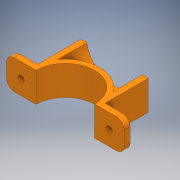
# Autodesk Inventor part: Motor Mount C-Clamp Base
Saved by Autodesk Inventor 2018 (Build 220112000, 112)
## iProperties
Created: 2018-01-11
Part Number: Motor Mount C-Clamp Base
Material: Generic
Document SubType Name: Modeling
Designer: Moochster
Density: 1 g/cm^3
Appearance: Orange
Author: Moochster
Autodesk Inventor part; units mm, degrees
ref_plane "YZ Plane" through (0, 0, 0) normal (1, 0, 0) x (0, 1, 0)
ref_plane "XY Plane" through (0, 0, 0) normal (0, 0, 1) x (1, 0, 0)
sketch "Sketch1" plane through (0, 0, 0) normal (0, 0, 1) x (1, 0, 0)
  arc A0 (14.865, 0) -> (-14.865, 0) centre (0, 0) ccw
  arc A1 (17.1039, 3) -> (-17.1039, 3) centre (0, 0) ccw
  line L0 (-17.1039, 3) -> (-29.865, 3)
  line L1 (-29.865, 3) -> (-29.865, 0)
  line L2 (-29.865, 0) -> (-14.865, 0)
  line L3 (14.865, 0) -> (29.865, 0)
  line L4 (29.865, 0) -> (29.865, 3)
  line L5 (29.865, 3) -> (17.1039, 3)
  dimension "d0" = 3
  dimension "d1" = 14.865
  dimension "d2" = 2.5
  dimension "d3" = 15
  constraints: 12 end point, 4 horizontal, 4 point on circle, 3 horizontal alignment, 2 centre point, 2 coincident, 2 perpendicular, 1 collinear, 1 concentric
  measures "d0" distance of L3.end L4.end
  measures "d1" radius of A0
  measures "d2" radial gap between concentric circles of A0 A1
  measures "d3" distance of L3.start L3.end
extrude "Extrusion1" add sketch "Sketch1" along normal blind 15
sketch "Sketch2" plane through (-29.865, 0, 0) normal (0, -1, 0) x (1, 0, 0)
  line L0 (0, 15) -> (15, 15) projected
  line L1 (0, 0) -> (0, 15) projected
  point P0 (29.865, 0)
  point P1 (7.5, 7.5)
  point P2 (7.5, 15)
  point P3 (0, 7.5)
  constraints: 2 midpoint, 1 horizontal alignment, 1 vertical alignment
hole "Hole1" at (-22.365, 0, 7.5) direction (0, 1, 0) diameter 3 end through all
mirror "Mirror1" about plane through (0, 0, 0) normal (1, 0, 0) of "Hole1"
ref_plane "Work Plane1" through (0, 25, 0) normal (0, 1, 0) x (-1, 0, 0)
sketch "Sketch3" plane through (0, 25, 0) normal (0, 1, 0) x (-1, 0, 0)
  line L0 (-17.1039, 0) -> (17.1039, 0) projected
  line L1 (-17.1039, 0) -> (-17.1039, 15) projected
  line L2 (17.1039, 0) -> (17.1039, 15) projected
  line L3 (-17.1039, 15) -> (-14.1039, 15)
  line L4 (17.1039, 15) -> (14.1039, 15)
  arc A0 (-14.1039, 15) -> (14.1039, 15) centre (0, 17.2883) ccw
  point P0 (0, 0)
  point P1 (0, 3)
  dimension "d14" = 3
  dimension "d15" = 3
  dimension "d16" = 3
  constraints: 4 end point, 3 point on circle, 2 horizontal, 1 centre point
  measures "d14" distance of L1.end L3.end
  measures "d15" distance of L2.end L4.end
  measures "d16" distance from line of L0 point (0, 3)
extrude "Extrusion2" add sketch "Sketch3" against normal up to next
fillet "Fillet1" radius 4 4 edges at (-29.865, 1.5, 15) (-29.865, 1.5, 0) (29.865, 1.5, 0) (29.865, 1.5, 15)
body "Solid1"
